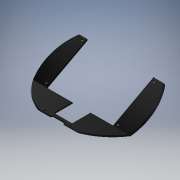
# Autodesk Inventor part: vd
Saved by Autodesk Inventor 2017 (Build 210142000, 142)
## iProperties
Part Number: vd
Material: Genérico
Document SubType Name: Modeling
Designer: Roberto
Density: 1 g/cm^3
Appearance: Valor por defecto
Author: Roberto
Autodesk Inventor part; units mm, degrees
ref_plane "Plano de trabajo1" through (-6.9595, -0.404, -3.0761) normal (0.0001326, 0.4716523, -0.8817846) x (-1, -0.0001499, -0.0002305)
sketch "Boceto1" plane through (-6.9595, -0.404, -3.0761) normal (0.0001326, 0.4716523, -0.8817846) x (-1, -0.0001499, -0.0002305)
  ellipse E0 centre (0.3242, 0.3023) end of major axis (0.3242, 0.4273) minor radius 0.125 projected
  ellipse E1 centre (0.3265, -4.7977) end of major axis (0.3265, -4.9227) minor radius 0.125 projected
  line L0 (-0.0484, -5.1729) -> (0.7516, -5.1725) projected
  line L1 (0.7516, -5.1725) -> (0.7491, 0.6275) projected
  line L2 (0.7491, 0.6275) -> (-0.0509, 0.6271) projected
  line L3 (-0.0484, -5.1729) -> (-0.0509, 0.6271) projected
  line L4 (0, -5.15) -> (0, 0.6) projected
  line L5 (-9.1491, -5.0234) -> (-9.1491, -5.1751) projected
  line L6 (-8.3491, -5.1749) -> (-9.1491, -5.1751) projected
  line L7 (-8.3491, -5.1749) -> (-8.3491, -5.15) projected
  line L8 (-8.3491, -5.15) -> (-8.9, -5.15) projected
  arc A0 (-9.05, -5) -> (-8.9, -5.15) centre (-8.9, -5) ccw projected
  line L9 (-9.05, -5) -> (-9.05, -4.7) projected
  arc A1 (-8.9, -4.55) -> (-9.05, -4.7) centre (-8.9, -4.7) ccw projected
  line L10 (-8.9, -4.55) -> (-8.4012, -4.55) projected
  line L11 (-8.4012, -4.55) -> (-8.4012, 0) projected
  line L12 (-8.4012, 0) -> (-8.9012, 0) projected
  arc A2 (-9.0512, 0.15) -> (-8.9012, 0) centre (-8.9012, 0.15) ccw projected
  line L13 (-9.0512, 0.15) -> (-9.0512, 0.45) projected
  arc A3 (-8.9012, 0.6) -> (-9.0512, 0.45) centre (-8.9012, 0.45) ccw projected
  line L14 (-8.9012, 0.6) -> (-8.3501, 0.6) projected
  line L15 (-8.3501, 0.6) -> (-8.3501, 0.6251) projected
  line L16 (-9.1501, 0.6249) -> (-8.3501, 0.6251) projected
  line L17 (-9.1491, -5.022) -> (-9.1501, 0.6249) projected
  line L18 (-9.1491, -5.0234) -> (-9.1491, -5.022) projected
  line L19 (-8.4012, 0.6) -> (-8.4012, -5.15) projected
  circle A4 centre (-8.725, 0.3) radius 0.125 projected
  circle A5 centre (-8.725, -4.85) radius 0.125 projected
  line L20 (-8.4012, -4.55) -> (-8.4012, 0) projected
  point P0 (-6.9603, 1.8054)
  constraints: 2 other
extrude "Extrusión1" add sketch "Boceto1" along normal blind 0.2
sketch "Boceto2" plane through (2.1908, -4.8309, -5.4426) normal (1, 0, 0.0001504) x (0.0001326, 0.4716523, -0.8817846)
  line L0 (0, 5.6469) -> (0, 0) projected
  line L1 (0, 0) -> (0.2, 0) projected
  line L2 (0.2, 5.6469) -> (0.2, 0) projected
  line L3 (0, 5.6469) -> (0.2, 5.6469) projected
  point P0 (-2.521, 6.827)
extrude "Extrusión2" add sketch "Boceto2" along normal blind 2
sketch "Boceto3" plane through (-7.7099, -4.9651, -5.5159) normal (-1, 0.000238, -0.0000231) x (-0.0001326, -0.4716523, 0.8817846)
  line L0 (0, 0) -> (0, 5.8) projected
  line L1 (0, 5.8) -> (-0.2, 5.8) projected
  line L2 (-0.2, 0) -> (-0.2, 5.8) projected
  line L3 (0, 0) -> (-0.2, 0) projected
  point P0 (2.521, 6.9813)
extrude "Extrusión3" add sketch "Boceto3" along normal blind 2
ref_plane "Plano de trabajo2" through (0.246, 3.4751, 0.2232) normal (0, 0, 1) x (1, 0, 0)
ref_plane "Plano de trabajo3" through (0.246, 3.4751, 0.1232) normal (0, 0, 1) x (1, 0, 0)
ref_plane "Plano de trabajo4" through (-1.3605, -7.2653, -8.5981) normal (0.0024365, 0.0000046, -0.999997) x (-0.0026205, 0.9999966, -0.0000018)
sketch "Boceto7" plane through (-1.3605, -7.2653, -8.5981) normal (0.0024365, 0.0000046, -0.999997) x (-0.0026205, 0.9999966, -0.0000018)
  line L0 (7.3744, -9.3505) -> (7.3172, -9.1132)
  line L1 (10.6651, -8.4624) -> (7.3172, -9.1132)
  line L2 (7.3172, -9.1132) -> (10.6651, -8.4624)
  line L3 (10.6651, -8.7392) -> (10.6651, -8.4336)
  line L4 (10.6651, -8.7392) -> (10.6651, -8.4336)
  line L5 (10.6651, -8.4624) -> (10.6651, -8.7392)
  line L6 (7.3744, -9.3505) -> (10.6651, -8.7392)
  line L7 (7.3744, -9.3505) -> (10.6651, -8.7392)
  line L8 (10.6651, -8.7392) -> (10.6651, 6.2608)
  arc A0 (-0.8965, -4.8887) -> (7.3744, -9.3505) centre (6.5114, -1.0534) ccw
  arc A1 (-1.7199, -1.2392) -> (-0.6466, -4.8446) centre (7.8839, -0.3428) ccw
  line L9 (-1.9628, -1.2392) -> (-1.7199, -1.2392)
  arc A2 (-1.9628, -1.2392) -> (-0.8965, -4.8887) centre (7.8839, -0.3428) ccw
  arc A3 (-0.6818, -4.7774) -> (7.3172, -9.1132) centre (6.5114, -1.0534) ccw
  line L10 (10.6651, -1.2392) -> (-7.9457, -1.2392)
  line L11 (7.3744, -9.3505) -> (7.3172, -9.1132)
  line L12 (10.6651, -8.4624) -> (7.3172, -9.1132)
  line L13 (7.3172, -9.1132) -> (10.6651, -8.4624)
  line L14 (10.6651, -8.7392) -> (10.6651, -8.4336)
  line L15 (10.6651, -8.7392) -> (10.6651, -8.4336)
  line L16 (10.6651, -8.4624) -> (10.6651, -8.7392)
  line L17 (7.3744, -9.3505) -> (10.6651, -8.7392)
  line L18 (7.3744, -9.3505) -> (10.6651, -8.7392)
  line L19 (10.6651, -8.7392) -> (10.6651, 6.2608)
  arc A4 (-0.8965, -4.8887) -> (7.3744, -9.3505) centre (6.5114, -1.0534) ccw
  arc A5 (-1.7199, -1.2392) -> (-0.6466, -4.8446) centre (7.8839, -0.3428) ccw
  line L20 (-1.9628, -1.2392) -> (-1.7199, -1.2392)
  arc A6 (-1.9628, -1.2392) -> (-0.8965, -4.8887) centre (7.8839, -0.3428) ccw
  arc A7 (-0.6818, -4.7774) -> (7.3172, -9.1132) centre (6.5114, -1.0534) ccw
  line L21 (10.6651, -1.2392) -> (-7.9457, -1.2392)
  line L22 (-1.9628, -1.2392) -> (-1.9628, -13.6721)
  line L23 (-1.9628, -13.6721) -> (10.6651, -13.4962)
  line L24 (10.6651, -8.4624) -> (10.6651, -13.4962)
  point P0 (7.2616, 1.4005)
  dimension "d18" = 15
  dimension "d19" = 15
  constraints: 50 end point, 22 point on circle, 8 centre point, 6 collinear, 4 coincident, 2 midpoint, 1 vertical
  measures "d18" distance of L8.start L8.end
  measures "d19" distance of L19.start L19.end
revolve "Revolución3" cut sketch "Boceto7" angle 360 about axis through (-2.6276, 3.3966, -8.6011) along (0.0026205, -0.9999966, 0.0000018) contours A0 A2 L9 A1 A3 L0 | L0 L1 L3 L6 | L6 L24 L23 L22 A2 A0
ref_plane "Plano de trabajo5" through (-1.3661, -7.2653, -6.2981) normal (0.9999936, 0.0026205, 0.0024365) x (0.0024365, 0.0000046, -0.999997)
sketch "Boceto8" plane through (-1.3661, -7.2653, -6.2981) normal (0.9999936, 0.0026205, 0.0024365) x (0.0024365, 0.0000046, -0.999997)
  line L0 (-0.7998, 2.3193) -> (-0.6238, 2.4141) projected
  line L1 (-3.2459, 7.3172) -> (-3.4725, 7.3172) projected
  line L2 (-0.6238, 2.4141) -> (-0.6238, 2.3193)
  line L3 (-0.6238, 2.3193) -> (-0.6238, -0.5167)
  line L4 (-0.7998, 2.3193) -> (-0.7998, -0.5167)
  line L5 (-0.7998, -0.5167) -> (-0.6238, -0.5167)
  line L6 (-0.788, 2.314) -> (-3.5, 7.3842) projected
  line L7 (-0.7998, 2.3193) -> (-0.6238, 2.4141)
  point P0 (-6.2947, 7.2616)
  constraints: 10 end point, 1 perpendicular, 1 vertical, 2 other
extrude "Extrusión5" add sketch "Boceto8" along normal mid plane 15
sketch "Boceto9" plane through (2.1908, -4.8309, -5.4426) normal (1, -0.0000625, 0.0001169) x (0.0001326, 0.4716523, -0.8817846)
  line L0 (0.1915, -0.1149) -> (0.171, -0.1531) projected
  line L1 (0.171, -0.1531) -> (0.2, -0.1531) projected
  line L2 (0.2, 0) -> (0.2, -0.1531) projected
  line L3 (0, 0) -> (0.2, 0) projected
  line L4 (0, 0) -> (0, -0.1154) projected
  line L5 (0, -0.1154) -> (0.1915, -0.1149) projected
  point P0 (-2.521, 6.8268)
extrude "Extrusión6" add sketch "Boceto9" along normal blind 4.5
sketch "Boceto10" plane through (-1.3605, -7.2653, -8.5981) normal (0.0024365, 0.0000046, -0.999997) x (-0.0026205, 0.9999966, -0.0000018)
  arc A0 (-1.9628, -1.2392) -> (-0.8965, -4.8887) centre (7.8839, -0.3428) ccw
  line L0 (-1.9628, -1.2392) -> (-1.7199, -1.2392)
  arc A1 (-1.7199, -1.2392) -> (-0.6466, -4.8446) centre (7.8839, -0.3428) ccw
  line L1 (7.3744, -9.3505) -> (7.3172, -9.1132)
  line L2 (10.6651, -1.2392) -> (-7.9457, -1.2392)
  arc A2 (-0.8965, -4.8887) -> (7.3744, -9.3505) centre (6.5114, -1.0534) ccw
  arc A3 (-0.6818, -4.7774) -> (7.3172, -9.1132) centre (6.5114, -1.0534) ccw
  line L3 (10.6651, -8.7392) -> (10.6651, 6.2608)
  line L4 (10.6651, -8.4624) -> (7.3172, -9.1132)
  line L5 (7.3172, -9.1132) -> (10.6651, -8.4624)
  line L6 (7.3744, -9.3505) -> (10.6651, -8.7392)
  line L7 (7.3744, -9.3505) -> (10.6651, -8.7392)
  line L8 (10.6651, -8.7392) -> (10.6651, -8.4336)
  line L9 (10.6651, -8.7392) -> (10.6651, -8.4336)
  line L10 (10.6651, -8.4624) -> (10.6651, -8.7392)
  arc A4 (-1.9628, -1.2392) -> (-0.8965, -4.8887) centre (7.8839, -0.3428) ccw
  line L11 (-1.9628, -1.2392) -> (-1.7199, -1.2392)
  arc A5 (-1.7199, -1.2392) -> (-0.6466, -4.8446) centre (7.8839, -0.3428) ccw
  line L12 (7.3744, -9.3505) -> (7.3172, -9.1132)
  line L13 (10.6651, -1.2392) -> (-7.9457, -1.2392)
  arc A6 (-0.8965, -4.8887) -> (7.3744, -9.3505) centre (6.5114, -1.0534) ccw
  arc A7 (-0.6818, -4.7774) -> (7.3172, -9.1132) centre (6.5114, -1.0534) ccw
  line L14 (10.6651, -8.7392) -> (10.6651, 6.2608)
  line L15 (10.6651, -8.4624) -> (7.3172, -9.1132)
  line L16 (7.3172, -9.1132) -> (10.6651, -8.4624)
  line L17 (7.3744, -9.3505) -> (10.6651, -8.7392)
  line L18 (7.3744, -9.3505) -> (10.6651, -8.7392)
  line L19 (10.6651, -8.7392) -> (10.6651, -8.4336)
  line L20 (10.6651, -8.7392) -> (10.6651, -8.4336)
  line L21 (10.6651, -8.4624) -> (10.6651, -8.7392)
  line L22 (-1.9628, -1.2392) -> (-1.9628, -13.6721)
  line L23 (-1.9628, -13.6721) -> (10.6651, -13.4962)
  line L24 (10.6651, -8.4624) -> (10.6651, -13.4962)
  arc A8 (-1.9628, -1.2392) -> (-0.8965, -4.8887) centre (7.8839, -0.3428) ccw
  line L25 (-1.9628, -1.2392) -> (-1.7199, -1.2392)
  arc A9 (-1.7199, -1.2392) -> (-0.6466, -4.8446) centre (7.8839, -0.3428) ccw
  line L26 (7.3744, -9.3505) -> (7.3172, -9.1132)
  line L27 (10.6651, -1.2392) -> (-7.9457, -1.2392)
  arc A10 (-0.8965, -4.8887) -> (7.3744, -9.3505) centre (6.5114, -1.0534) ccw
  arc A11 (-0.6818, -4.7774) -> (7.3172, -9.1132) centre (6.5114, -1.0534) ccw
  line L28 (10.6651, -8.7392) -> (10.6651, 6.2608)
  line L29 (10.6651, -8.4624) -> (7.3172, -9.1132)
  line L30 (7.3172, -9.1132) -> (10.6651, -8.4624)
  line L31 (7.3744, -9.3505) -> (10.6651, -8.7392)
  line L32 (7.3744, -9.3505) -> (10.6651, -8.7392)
  line L33 (10.6651, -8.7392) -> (10.6651, -8.4336)
  line L34 (10.6651, -8.7392) -> (10.6651, -8.4336)
  line L35 (10.6651, -8.4624) -> (10.6651, -8.7392)
  arc A12 (-1.9628, -1.2392) -> (-0.8965, -4.8887) centre (7.8839, -0.3428) ccw
  line L36 (-1.9628, -1.2392) -> (-1.7199, -1.2392)
  arc A13 (-1.7199, -1.2392) -> (-0.6466, -4.8446) centre (7.8839, -0.3428) ccw
  line L37 (7.3744, -9.3505) -> (7.3172, -9.1132)
  line L38 (10.6651, -1.2392) -> (-7.9457, -1.2392)
  arc A14 (-0.8965, -4.8887) -> (7.3744, -9.3505) centre (6.5114, -1.0534) ccw
  arc A15 (-0.6818, -4.7774) -> (7.3172, -9.1132) centre (6.5114, -1.0534) ccw
  line L39 (10.6651, -8.7392) -> (10.6651, 6.2608)
  line L40 (10.6651, -8.4624) -> (7.3172, -9.1132)
  line L41 (7.3172, -9.1132) -> (10.6651, -8.4624)
  line L42 (7.3744, -9.3505) -> (10.6651, -8.7392)
  line L43 (7.3744, -9.3505) -> (10.6651, -8.7392)
  line L44 (10.6651, -8.7392) -> (10.6651, -8.4336)
  line L45 (10.6651, -8.7392) -> (10.6651, -8.4336)
  line L46 (10.6651, -8.4624) -> (10.6651, -8.7392)
  line L47 (-1.9628, -1.2392) -> (-1.9628, -13.6721)
  line L48 (-1.9628, -13.6721) -> (10.6651, -13.4962)
  line L49 (10.6651, -8.4624) -> (10.6651, -13.4962)
  arc A16 (-1.9628, -1.2392) -> (-0.8965, -4.8887) centre (7.8839, -0.3428) ccw
  line L50 (-1.9628, -1.2392) -> (-1.7199, -1.2392)
  arc A17 (-1.7199, -1.2392) -> (-0.6466, -4.8446) centre (7.8839, -0.3428) ccw
  line L51 (7.3744, -9.3505) -> (7.3172, -9.1132)
  line L52 (10.6651, -1.2392) -> (-7.9457, -1.2392)
  arc A18 (-0.8965, -4.8887) -> (7.3744, -9.3505) centre (6.5114, -1.0534) ccw
  arc A19 (-0.6818, -4.7774) -> (7.3172, -9.1132) centre (6.5114, -1.0534) ccw
  line L53 (10.6651, -8.7392) -> (10.6651, 6.2608)
  line L54 (10.6651, -8.4624) -> (7.3172, -9.1132)
  line L55 (7.3172, -9.1132) -> (10.6651, -8.4624)
  line L56 (7.3744, -9.3505) -> (10.6651, -8.7392)
  line L57 (7.3744, -9.3505) -> (10.6651, -8.7392)
  line L58 (10.6651, -8.7392) -> (10.6651, -8.4336)
  line L59 (10.6651, -8.7392) -> (10.6651, -8.4336)
  line L60 (10.6651, -8.4624) -> (10.6651, -8.7392)
  arc A20 (-1.9628, -1.2392) -> (-0.8965, -4.8887) centre (7.8839, -0.3428) ccw
  line L61 (-1.9628, -1.2392) -> (-1.7199, -1.2392)
  arc A21 (-1.7199, -1.2392) -> (-0.6466, -4.8446) centre (7.8839, -0.3428) ccw
  line L62 (7.3744, -9.3505) -> (7.3172, -9.1132)
  line L63 (10.6651, -1.2392) -> (-7.9457, -1.2392)
  arc A22 (-0.8965, -4.8887) -> (7.3744, -9.3505) centre (6.5114, -1.0534) ccw
  arc A23 (-0.6818, -4.7774) -> (7.3172, -9.1132) centre (6.5114, -1.0534) ccw
  line L64 (10.6651, -8.7392) -> (10.6651, 6.2608)
  line L65 (10.6651, -8.4624) -> (7.3172, -9.1132)
  line L66 (7.3172, -9.1132) -> (10.6651, -8.4624)
  line L67 (7.3744, -9.3505) -> (10.6651, -8.7392)
  line L68 (7.3744, -9.3505) -> (10.6651, -8.7392)
  line L69 (10.6651, -8.7392) -> (10.6651, -8.4336)
  line L70 (10.6651, -8.7392) -> (10.6651, -8.4336)
  line L71 (10.6651, -8.4624) -> (10.6651, -8.7392)
  line L72 (-1.9628, -1.2392) -> (-1.9628, -13.6721)
  line L73 (-1.9628, -13.6721) -> (10.6651, -13.4962)
  line L74 (10.6651, -8.4624) -> (10.6651, -13.4962)
  point P0 (7.2616, 1.4005)
  point P1 (7.2616, 1.4005)
  point P2 (7.2616, 1.4005)
  point P3 (7.2616, 1.4005)
  dimension "d25" = 15
  dimension "d26" = 15
  dimension "d27" = 15
  dimension "d28" = 15
  dimension "d29" = 15
  dimension "d30" = 15
  constraints: 150 end point, 66 point on circle, 24 centre point, 18 collinear, 12 coincident, 6 midpoint, 3 vertical
  measures "d25" distance of L8.start L3.end
  measures "d26" distance of L19.start L14.end
  measures "d27" distance of L33.start L28.end
  measures "d28" distance of L44.start L39.end
  measures "d29" distance of L58.start L53.end
  measures "d30" distance of L69.start L64.end
revolve "Revolución4" cut sketch "Boceto10" angle 360 about axis through (-2.6276, 3.3966, -8.6011) along (0.0026205, -0.9999966, 0.0000018) contours L0 A1 A3 L1 A2 A0 | A0 A2 L6 L24 L23 L22 | L1 L4 L3 L6
sketch "Boceto11" plane through (1.4429, -4.8438, -5.6674) normal (0.0024365, 0.0000046, -0.999997) x (-0.9999936, -0.0026205, -0.0024365)
  line L0 (2.9669, -0.5141) -> (2.9669, 0.0859) projected
  line L1 (2.9669, 0.0859) -> (2.8169, 0.0859) projected
  line L2 (2.8169, 0.0859) -> (2.8169, -2.4141) projected
  line L3 (2.8169, -2.4141) -> (5.1169, -2.4141) projected
  line L4 (5.1169, -2.4141) -> (5.1169, 0.0859) projected
  line L5 (5.1169, 0.0859) -> (4.9669, 0.0859) projected
  line L6 (4.9669, 0.0859) -> (4.9669, -0.5141) projected
  line L7 (4.9669, -0.5141) -> (2.9669, -0.5141) projected
  circle A0 centre (4.9369, -0.9141) radius 0.1 projected
  circle A1 centre (4.9369, -2.2141) radius 0.1 projected
  circle A2 centre (2.9969, -0.9141) radius 0.1 projected
  circle A3 centre (2.9969, -2.2141) radius 0.1 projected
  line L8 (4.9669, -0.5141) -> (4.9669, 0.0859) projected
  line L9 (4.9669, 0.0859) -> (2.9669, 0.0859) projected
  line L10 (2.9669, 0.0859) -> (2.9669, -0.5141) projected
  line L11 (2.9669, -0.5141) -> (4.9669, -0.5141) projected
  point P0 (1.4164, 4.8476)
extrude "Extrusión7" cut sketch "Boceto11" against normal blind 4.5 contours L7 L6 L5 L4 L3 L2 L1 L0 | L0 L9 L6 L7 | A0 | A1 | A2 | A3
sketch "Boceto12" plane through (-6.9098, -4.8734, -5.6878) normal (0.0024365, 0.0000046, -0.999997) x (-0.9999959, 0.0015288, -0.0024364)
  circle A0 centre (-2.3896, -2.6965) radius 0.1 projected
  line L0 (-3.2359, 0.0211) -> (-3.2459, -2.393) projected
  line L1 (-3.2459, -2.393) -> (-5.5459, -2.3834) projected
  line L2 (-5.5459, -2.3834) -> (-5.5359, 0.0306) projected
  line L3 (-8.3527, 0.0423) -> (-5.5359, 0.0306) projected
  line L4 (-8.3528, 0.0301) -> (-8.3527, 0.0423) projected
  line L5 (-8.3007, 0.0301) -> (-8.3528, 0.0301) projected
  line L6 (-8.3007, 0.0018) -> (-8.3007, 0.0301) projected
  line L7 (-9.1007, 0.002) -> (-8.3007, 0.0018) projected
  line L8 (-9.1006, 0.0454) -> (-9.1007, 0.002) projected
  line L9 (-9.1006, 0.0454) -> (-10.4343, 0.0457) projected
  line L10 (-1.8176, -2.9156) -> (-6.8001, -2.8949) projected
  line L11 (0, 0) -> (1.8442, 0) projected
  line L12 (0, 0.0077) -> (0, 0) projected
  line L13 (-3.2359, 0.0211) -> (0, 0.0077) projected
  circle A1 centre (-5.6896, -2.6828) radius 0.1 projected
  line L14 (-3.3848, -3.0867) -> (-4.9848, -3.0791) projected
  line L15 (-2.0403, -2.9146) -> (-6.5774, -2.8958) projected
  line L16 (-3.3841, -2.9091) -> (-3.3832, -2.7091)
  line L17 (-3.3832, -2.7091) -> (-4.9848, -2.7024)
  line L18 (-4.9848, -2.9024) -> (-4.9848, -2.7024)
  line L19 (-3.3841, -2.9091) -> (-4.9848, -2.9024)
  point P0 (-6.9162, 4.884)
  constraints: 8 end point, 2 point on line, 1 collinear, 1 perpendicular, 1 vertical, 2 other
extrude "Extrusión8" cut sketch "Boceto12" against normal blind 4.5
